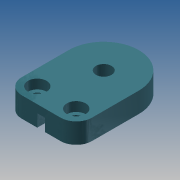
# Autodesk Inventor part: belt tensioner
Saved by Autodesk Inventor 2013 (Build 170138000, 138)
## iProperties
Created: 2017-04-01
Part Number: belt tensioner
Material: Generic
Document SubType Name: Modeling
Designer: employee
Density: 1 g/cm^3
Author: employee
Autodesk Inventor part; units mm, degrees
ref_plane "YZ Plane" through (0, 0, 0) normal (1, 0, 0) x (0, 1, 0)
ref_plane "XZ Plane" through (0, 0, 0) normal (0, 1, 0) x (-1, 0, 0)
ref_plane "XY Plane" through (0, 0, 0) normal (0, 0, 1) x (1, 0, 0)
sketch "Sketch1" plane through (0, 0, 0) normal (0, 0, 1) x (1, 0, 0)
  line L0 (-1.25, 0) -> (1.25, 0)
  line L1 (-1.25, 0) -> (-1.25, 7)
  arc A0 (-1.25, 7) -> (-4.625, 13.5276) centre (-9.25, 7) ccw
  arc A1 (4.625, 13.5276) -> (-4.625, 13.5276) centre (0, 20.0552) ccw
  arc A2 (4.625, 13.5276) -> (1.25, 7) centre (9.25, 7) ccw
  line L2 (1.25, 7) -> (1.25, 0)
  circle A3 centre (0, 20.0552) radius 6.5
  line L3 (-1.25, 0) -> (-11.25, 0)
  line L4 (-11.25, 0) -> (-11.25, 31.3052)
  line L5 (-11.25, 31.3052) -> (11.25, 31.3052)
  line L6 (11.25, 31.3052) -> (11.25, 0)
  line L7 (11.25, 0) -> (1.25, 0)
  point P0 (0, 0)
  point P1 (0, 0)
  dimension "d0" = 2.5
  dimension "d3" = 7
  dimension "d4" = 1.5
  dimension "d15" = 10
  dimension "d23" = 11.25
  dimension "d24" = 8
  constraints: 16 end point, 6 point on circle, 4 centre point, 4 perpendicular, 4 tangent, 2 coincident, 2 equal length, 2 equal radius, 2 parallel, 1 collinear, 1 horizontal, 1 midpoint
  measures "d0" distance of L0.start L0.end
  measures "d3" distance of L2.start L0.end
  measures "d4" radial gap between concentric circles of A1 A3
  measures "d15" distance between parallel lines of L4 L1
  measures "d23" distance from line of L5 A1.centre
  measures "d24" radius of A1
extrude "Extrusion1" add sketch "Sketch1" along normal blind 6.5 contours L3 L4 L5 L6 L7 L2 A2 A1 A0 L1 | A3
fillet "Fillet1" radius 11.25 2 edges at (11.25, 31.3052, 3.25) (-11.25, 31.3052, 3.25)
sketch "Sketch2" plane through (0, 0, 6.5) normal (0, 0, 1) x (1, 0, 0)
  line L0 (-1.25, 0) -> (-1.25, 7) projected
  arc A0 (-1.25, 7) -> (-4.625, 13.5276) centre (-9.25, 7) ccw projected
  arc A1 (4.625, 13.5276) -> (-4.625, 13.5276) centre (0, 20.0552) ccw projected
  arc A2 (4.625, 13.5276) -> (1.25, 7) centre (9.25, 7) ccw projected
  line L1 (1.25, 7) -> (1.25, 0) projected
  line L2 (11.25, 0) -> (11.25, 20.0552) projected
  line L3 (-1.25, 0) -> (1.25, 0)
  point P0 (0, 0)
  constraints: 2 end point, 1 perpendicular
extrude "Extrusion2" add sketch "Sketch2" against normal blind 2.5
sketch "Sketch3" plane through (0, 0, 0) normal (0, 0, -1) x (-1, 0, 0)
  line L0 (-1.25, 0) -> (-11.25, 0) projected
  line L1 (11.25, 0) -> (1.25, 0) projected
  circle A0 centre (-6.25, 5) radius 1.75
  circle A1 centre (6.25, 5) radius 1.75
  point P0 (0, 0)
  point P1 (-1.25, 22.4355)
  point P2 (-6.25, 0)
  point P3 (6.25, 0)
  dimension "d13" = 5
  dimension "d14" = 3.5
  constraints: 2 centre point, 2 midpoint, 2 vertical alignment, 1 equal radius, 1 horizontal alignment
  measures "d13" distance from line of A0.centre L0
  measures "d14" diameter of A0
extrude "Extrusion3" cut sketch "Sketch3" against normal through all
sketch "Sketch4" plane through (0, 0, 6.5) normal (0, 0, 1) x (1, 0, 0)
  circle A0 centre (6.25, 5) radius 1.75 projected
  circle A1 centre (-6.25, 5) radius 1.75 projected
  circle A2 centre (-6.25, 5) radius 3
  circle A3 centre (6.25, 5) radius 3
  point P0 (0, 0)
  dimension "d19" = 6
  constraints: 2 centre point, 2 coincident, 1 equal radius
  measures "d19" diameter of A2
extrude "Extrusion4" cut sketch "Sketch4" against normal blind 3
fillet "Fillet2" radius 5 2 edges at (-11.25, 0, 3.25) (11.25, 0, 3.25)
sketch "Sketch5" plane through (0, 0, 6.5) normal (0, 0, 1) x (1, 0, 0)
  arc A0 (11.25, 20.0552) -> (-11.25, 20.0552) centre (0, 20.0552) ccw projected
  circle A1 centre (0, 20.0552) radius 2.5
  point P0 (0, 0)
  dimension "d26" = 5
  constraints: 1 centre point, 1 coincident
  measures "d26" diameter of A1
extrude "Extrusion5" cut sketch "Sketch5" against normal through all
equation "\"d9\" = d16"
equation "\"d16\" = 11.25"
body "Solid1"
